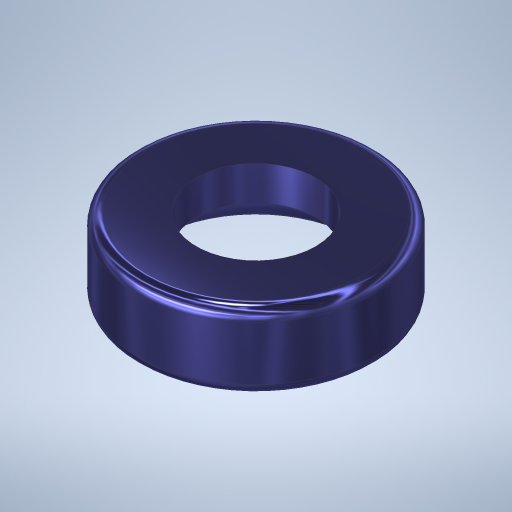
# Autodesk Inventor part: Pillow Ball Bushing
Saved by Autodesk Inventor 2023.1 (Build 271208000, 208)
## iProperties
Created: 2019-11-30
Part Number: Pillow Ball Bushing
Material: Generic
Document SubType Name: Modeling
Designer: Jopa
Density: 1 g/cm^3
Appearance: Default
Author: Jopa
Autodesk Inventor part; units mm, degrees
ref_plane "YZ Plane" through (0, 0, 0) normal (1, 0, 0) x (0, 1, 0)
ref_plane "XZ Plane" through (0, 0, 0) normal (0, 1, 0) x (-1, 0, 0)
ref_plane "XY Plane" through (0, 0, 0) normal (0, 0, 1) x (1, 0, 0)
sketch "Sketch1" plane through (0, 0, 0) normal (0, 0, 1) x (1, 0, 0)
  line L0 (0, -0.996467) -> (0, 5.9788) construction
  line L1 (-0.996467, 0) -> (5.9788, 0) construction
  line L2 (4.1275, 0) -> (4.1275, 4.7625)
  line L3 (4.1275, 4.7625) -> (0, 4.7625)
  line L4 (0, 4.7625) -> (0, 4.1275)
  arc A0 (4.1275, 0) -> (0, 4.1275) centre (0, 0) ccw
  point P0 (0, 0)
  dimension "d0" = 4.7625
  dimension "d1" = 4.1275
  dimension "d2" = 0.635
  dimension "d3" = 4.1275
  constraints: 6 end point, 3 point on line, 2 point on circle, 1 centre point, 1 horizontal, 1 vertical
  measures "d0" distance of L2.start L2.end
  measures "d1" distance of L2.end L3.end
  measures "d2" distance of L3.end L4.end
  measures "d3" radius of A0
sketch "Sketch1 outline for Revolution1" plane through (0, 0, 0) normal (0, 0, 1) x (1, 0, 0)
  arc A0 (0, 4.1275) -> (4.1275, 0) centre (0, 0) cw
  line L0 (0, 4.7625) -> (0, 4.1275)
  line L1 (4.1275, 4.7625) -> (0, 4.7625)
  line L2 (4.1275, 0) -> (4.1275, 4.7625)
revolve "Revolution1" add sketch "Sketch1 outline for Revolution1" angle 360 about axis through (0, -10, 0) along (0, 1, 0)
fillet "Fillet1" radius 0.381 2 edges at (-4.1275, 4.7625, 0) (-4.1275, 0, 0)
sketch "Sketch2" plane through (0, 4.7625, 0) normal (0, 1, 0) x (1, 0, 0)
  circle A0 centre (0, 0) radius 2.06375
  dimension "d6" = 4.1275
  constraints: 1 centre point, 1 coincident
  measures "d6" diameter of A0
sketch "Sketch2 outline for Extrusion1" plane through (0, 4.7625, 0) normal (0, 1, 0) x (1, 0, 0)
  circle A0 centre (0, 0) radius 2.06375
extrude "Extrusion1" cut sketch "Sketch2 outline for Extrusion1" along normal through all both and the other way through all
body "Solid1"
